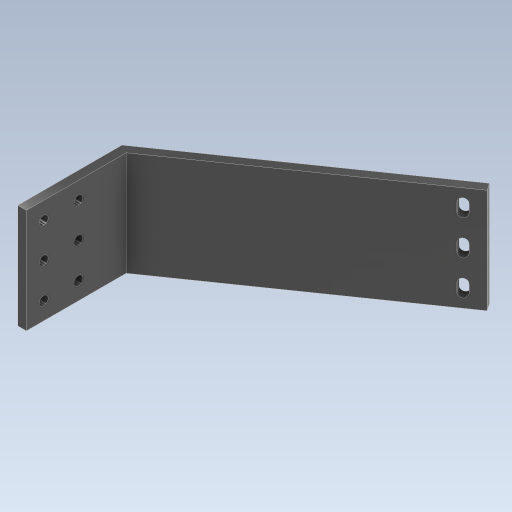
# Autodesk Inventor part: INDX_006_Funnel
Saved by Autodesk Inventor 2024 (Build 280153000, 153)
## iProperties
Created: 2024-08-09
Part Number: INDX_006_Funnel
Material: ABS Plastic
Document SubType Name: Modeling
Designer: Oscar
Density: 1.06 g/cm^3
Appearance: Dark Gray
Author: Oscar
Autodesk Inventor part; units mm, degrees
ref_plane "YZ Plane" through (0, 0, 0) normal (1, 0, 0) x (0, 1, 0)
ref_plane "XZ Plane" through (0, 0, 0) normal (0, 1, 0) x (-1, 0, 0)
ref_plane "XY Plane" through (0, 0, 0) normal (0, 0, 1) x (1, 0, 0)
sketch "Sketch1" plane through (0, 0, 0) normal (0, 1, 0) x (-1, 0, 0)
  line L0 (0, 0) -> (-6.35, 0)
  line L1 (-6.35, 0) -> (-6.35, -76.2)
  line L2 (-6.35, -76.2) -> (0, -76.2)
  line L3 (0, -76.2) -> (0, 0)
  line L4 (-6.35, -72.8797) -> (-161.925, -180.975)
  line L5 (-158.3017, -186.1898) -> (0, -76.2)
  line L6 (-158.3017, -186.1898) -> (-161.925, -180.975)
  point P0 (-6.35, -38.1)
  point P1 (-3.175, -76.2)
  point P2 (-6.35, -6.35)
  dimension "d9" = 6.35
  dimension "d10" = 76.2
  dimension "d30" = 6.35
  dimension "d31" = 6.35
  dimension "d32" = 155.575
  dimension "d33" = 174.625
  dimension "d53" = 6.35
  constraints: 14 end point, 3 parallel, 2 midpoint, 2 perpendicular, 1 horizontal, 1 point on line
  measures "d9" distance of L2.end L1.end
  measures "d10" distance of L1.end L0.end
  measures "d30" distance from line of L3 point (-6.35, -6.35)
  measures "d31" distance from line of L0 point (-6.35, -6.35)
  measures "d32" horizontal distance of point (-6.35, -6.35) L4.end
  measures "d33" vertical distance of point (-6.35, -6.35) L4.end
  measures "d53" distance between parallel lines of L5 L4
extrude "Extrusion1" add sketch "Sketch1" along normal blind 76.2
sketch "Sketch2" plane through (0, 0, -76.2) normal (-1, 0, 0) x (0, 0, 1)
  circle A0 centre (63.5, 12.7) radius 3.2639
  circle A1 centre (63.5, 38.1) radius 3.2639
  circle A2 centre (63.5, 63.5) radius 3.2639
  line L0 (0, 0) -> (0, 76.2) projected
  line L1 (0, 0) -> (76.2, 0) projected
  line L2 (76.2, 0) -> (76.2, 76.2) projected
  circle A3 centre (38.1, 63.5) radius 3.2639
  circle A4 centre (38.1, 38.1) radius 3.2639
  circle A5 centre (38.1, 12.7) radius 3.2639
  dimension "d18" = 6.5278
  dimension "d19" = 25.4
  dimension "d21" = 25.4
  dimension "d22" = 12.7
  dimension "d34" = 12.7
  dimension "d35" = 25.4
  dimension "d36" = 25.4
  dimension "d38" = 25.4
  constraints: 6 centre point, 5 equal radius, 4 vertical alignment, 1 horizontal alignment
  measures "d18" diameter of A0
  measures "d19" distance of A2.centre A1.centre
  measures "d21" distance of A1.centre A0.centre
  measures "d22" distance from line of L1 A0.centre
  measures "d34" distance from line of L2 A1.centre
  measures "d35" distance of A4.centre A5.centre
  measures "d36" distance of A3.centre A4.centre
  measures "d38" distance of A4.centre A1.centre
extrude "Extrusion2" cut sketch "Sketch2" against normal through all
sketch "Sketch4" plane through (161.925, 0, -180.975) normal (0.5706, 0, 0.8212) x (0.8212, 0, -0.5706)
  arc A0 (-9.525, 66.675) -> (-15.875, 66.675) centre (-12.7, 66.675) ccw
  arc A1 (-15.875, 60.325) -> (-9.525, 60.325) centre (-12.7, 60.325) ccw
  line L0 (-12.7, 76.4683) -> (-12.7, 0) construction
  line L1 (-189.4417, 0) -> (0, 0) construction
  line L2 (0, 0) -> (0, 76.2) construction
  line L3 (-15.875, 66.675) -> (-15.875, 60.325)
  line L4 (-9.525, 66.675) -> (-9.525, 60.325)
  arc A2 (-9.525, 41.275) -> (-15.875, 41.275) centre (-12.7, 41.275) ccw
  line L5 (-15.875, 41.275) -> (-15.875, 34.925)
  line L6 (-9.525, 41.275) -> (-9.525, 34.925)
  arc A3 (-15.875, 34.925) -> (-9.525, 34.925) centre (-12.7, 34.925) ccw
  arc A4 (-9.525, 15.875) -> (-15.875, 15.875) centre (-12.7, 15.875) ccw
  line L7 (-15.875, 15.875) -> (-15.875, 9.525)
  line L8 (-9.525, 15.875) -> (-9.525, 9.525)
  arc A5 (-15.875, 9.525) -> (-9.525, 9.525) centre (-12.7, 9.525) ccw
  point P0 (-236.2416, 0)
  point P1 (-182.3346, 0)
  point P2 (-9.525, 63.5)
  point P3 (-9.525, 38.1)
  point P4 (-9.525, 12.7)
  dimension "d39" = 6.35
  dimension "d40" = 6.35
  dimension "d41" = 6.35
  dimension "d42" = 12.7
  dimension "d43" = 63.5
  dimension "d46" = 25.4
  constraints: 14 end point, 12 point on circle, 6 centre point, 3 vertical, 2 point on line, 2 tangent, 1 midpoint, 1 parallel, 1 vertical alignment, 22 other
  measures "d39" diameter of A0
  measures "d40" diameter of A1
  measures "d41" distance of A0.centre A1.centre
  measures "d42" distance between parallel lines of L2 L0
  measures "d43" distance from line of L1 point (-9.525, 63.5)
  measures "d46" distance of A0.centre A2.centre
extrude "Extrusion3" cut sketch "Sketch4" against normal through all
body "Solid1"
